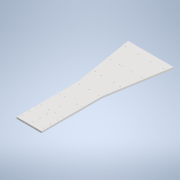
# Autodesk Inventor part: шея2,0
Saved by Autodesk Inventor 2020 (Build 240168000, 168)
## iProperties
Created: 2022-03-06
Part Number: шея2,0
Material: Типовые
Document SubType Name: Modeling
Designer: Администратор
Density: 1 g/cm^3
Appearance: По умолчанию
Author: Администратор
Autodesk Inventor part; units mm, degrees
ref_plane "YZ Plane" through (0, 0, 0) normal (1, 0, 0) x (0, 1, 0)
ref_plane "XZ Plane" through (0, 0, 0) normal (0, 1, 0) x (-1, 0, 0)
ref_plane "XY Plane" through (0, 0, 0) normal (0, 0, 1) x (1, 0, 0)
sketch "Эскиз1" plane through (0, 0, 0) normal (0, 1, 0) x (-1, 0, 0)
  line L0 (0, 0) -> (0, 458.3537) construction
  line L1 (0, 0) -> (0, -395.9132) construction
  line L2 (0, 0) -> (0, -1420) construction
  line L3 (0, -1420) -> (-240, -1420) construction
  line L4 (0, -1420) -> (240, -1420) construction
  line L5 (-240, -1420) -> (-11.5109, -68.1064) construction
  line L6 (-45, 13.7558) -> (45, 13.7558)
  line L7 (45, 13.7558) -> (45, -206.2442)
  line L8 (45, -206.2442) -> (-45, -206.2442) construction
  line L9 (-45, -206.2442) -> (-45, 13.7558)
  line L10 (-45, 13.7558) -> (45, -206.2442) construction
  line L11 (45, 13.7558) -> (-45, -206.2442) construction
  line L12 (-251.832, -1430) -> (-82.1831, -426.2442) construction
  line L13 (-45, -206.2442) -> (45, -206.2442) construction
  line L14 (45, -206.2442) -> (45, -426.2442) construction
  line L15 (45, -426.2442) -> (-45, -426.2442) construction
  line L16 (-45, -426.2442) -> (-45, -206.2442) construction
  line L17 (0, -426.2442) -> (-82.1831, -426.2442)
  line L18 (-82.1831, -426.2442) -> (-45, -206.2442)
  line L19 (0, -426.2442) -> (82.1831, -426.2442)
  line L20 (82.1831, -426.2442) -> (45, -206.2442)
  circle A0 centre (-11.5109, -68.1064) radius 1.5
  line L21 (-11.5109, -68.1064) -> (0, 0) construction
  circle A1 centre (-22.8432, -135.1555) radius 1.5
  circle A2 centre (-34.1754, -202.2045) radius 1.5
  circle A3 centre (-45.5077, -269.2536) radius 1.5
  circle A4 centre (-56.8399, -336.3027) radius 1.5
  circle A5 centre (-68.1721, -403.3518) radius 1.5
  circle A6 centre (11.5109, -68.1064) radius 1.5
  circle A7 centre (22.8432, -135.1555) radius 1.5
  circle A8 centre (34.1754, -202.2045) radius 1.5
  circle A9 centre (45.5077, -269.2536) radius 1.5
  circle A10 centre (56.8399, -336.3027) radius 1.5
  circle A11 centre (68.1721, -403.3518) radius 1.5
  line L22 (0, -96.2442) -> (0, -202.2045)
  circle A12 centre (0, -202.2045) radius 1.5
  circle A13 centre (0, -149.2045) radius 1.5
  circle A14 centre (0, -96.2045) radius 1.5
  point P0 (0, -96.2442)
  dimension "d16" = 240
  dimension "d17" = 180
  dimension "d18" = 1420
  dimension "d21" = 90
  dimension "d22" = 220
  dimension "d24" = 10
  dimension "d25" = 90
  dimension "d26" = 220
  dimension "d27" = 3
  dimension "d30" = 68
  dimension "d39" = 53
  constraints: 46 end point, 15 centre point, 7 symmetric about line, 5 horizontal, 4 midpoint, 4 parallel, 4 point on line, 4 vertical, 2 perpendicular, 1 coincident, 1 collinear, 21 other
  measures "d16" distance of L2.end L3.end
  measures "d17" angle of L3 L4
  measures "d18" distance of L0.start L2.end
  measures "d21" distance of L8.end L7.end
  measures "d22" distance of L6.end L7.end
  measures "d24" distance between parallel lines of L5 L12
  measures "d25" distance of L14.end L15.end
  measures "d26" distance of L13.end L14.end
  measures "d27" diameter of A0
  measures "d30" distance of L5.end A1.centre
  measures "d39" distance of A12.centre A13.centre
extrude "Выдавливание1" add sketch "Эскиз1" along normal blind 6 contours L6 L7 L20 L19 L17 L18 L9 | A12 | A13 L22 | L22 A13 | A14
extrude "Выдавливание2" cut sketch "Эскиз1" along normal blind 10 contours A12 | A13 L22 | L22 A13 | A14
sketch "Эскиз2" plane through (0, 6, 0) normal (0, 1, 0) x (1, 0, 0)
  circle A0 centre (-45.5077, 269.2536) radius 1.5 projected
  circle A1 centre (-56.8399, 336.3027) radius 1.5 projected
  circle A2 centre (0, 202.2045) radius 1.5 projected
  circle A3 centre (0, 149.2045) radius 1.5 projected
  circle A4 centre (0, 96.2045) radius 1.5 projected
  line L0 (45, 206.2442) -> (82.1831, 426.2442) projected
  line L1 (82.1831, 426.2442) -> (-82.1831, 426.2442) projected
  line L2 (-82.1831, 426.2442) -> (-45, 206.2442) projected
  line L3 (-45, 206.2442) -> (-45, -13.7558) projected
  line L4 (-45, -13.7558) -> (45, -13.7558) projected
  line L5 (45, -13.7558) -> (45, 206.2442) projected
  circle A5 centre (11.5109, 68.1064) radius 1.5 projected
  circle A6 centre (22.8432, 135.1555) radius 1.5 projected
  circle A7 centre (34.1754, 202.2045) radius 1.5 projected
  circle A8 centre (-11.5109, 68.1064) radius 1.5 projected
  circle A9 centre (-22.8432, 135.1555) radius 1.5 projected
  circle A10 centre (-34.1754, 202.2045) radius 1.5 projected
  circle A11 centre (45.5077, 269.2536) radius 1.5 projected
  circle A12 centre (56.8399, 336.3027) radius 1.5 projected
  circle A13 centre (68.1721, 403.3518) radius 1.5 projected
  circle A14 centre (-45.5077, 269.2536) radius 1.5 projected
  circle A15 centre (-56.8399, 336.3027) radius 1.5 projected
  circle A16 centre (-68.1721, 403.3518) radius 1.5 projected
  line L6 (-82.1831, 426.2442) -> (-45, 206.2442) projected
  line L7 (-55.6495, 269.2536) -> (55.6495, 269.2536)
  line L8 (45, 206.2442) -> (82.1831, 426.2442) projected
  line L9 (-66.9817, 336.3027) -> (66.9817, 336.3027)
  line L10 (-78.314, 403.3518) -> (78.314, 403.3518)
  circle A17 centre (-22.8432, 269.2536) radius 1.5
  circle A18 centre (22.8432, 269.2536) radius 1.5
  circle A19 centre (-22.8432, 336.3027) radius 1.5
  circle A20 centre (22.8432, 336.3027) radius 1.5
  circle A21 centre (-22.8432, 403.3518) radius 1.5
  circle A22 centre (22.8432, 403.3518) radius 1.5
  point P0 (0, 0)
  constraints: 12 point on line, 6 centre point, 6 end point, 2 parallel, 1 horizontal
extrude "Выдавливание3" cut sketch "Эскиз2" against normal blind 10 contours A17 L7 | L7 A17 | A18 L7 | L7 A18 | A19 L9 | L9 A19 | A21 L10 | L10 A21 | A20 L9 | L9 A20 | A22 L10 | L10 A22
sketch "Эскиз3" plane through (0, 6, 0) normal (0, 1, 0) x (1, 0, 0)
  circle A0 centre (-22.8432, 336.3027) radius 1.5 projected
  circle A1 centre (22.8432, 403.3518) radius 1.5 projected
  circle A2 centre (22.8432, 269.2536) radius 1.5 projected
  circle A3 centre (22.8432, 336.3027) radius 1.5 projected
  circle A4 centre (-22.8432, 403.3518) radius 1.5 projected
  circle A5 centre (-22.8432, 269.2536) radius 1.5 projected
  circle A6 centre (0, 202.2045) radius 1.5 projected
  circle A7 centre (0, 149.2045) radius 1.5 projected
  circle A8 centre (0, 96.2045) radius 1.5 projected
  line L0 (45, 206.2442) -> (82.1831, 426.2442) projected
  line L1 (82.1831, 426.2442) -> (-82.1831, 426.2442) projected
  line L2 (-82.1831, 426.2442) -> (-45, 206.2442) projected
  line L3 (-45, 206.2442) -> (-45, -13.7558) projected
  line L4 (-45, -13.7558) -> (45, -13.7558) projected
  line L5 (45, -13.7558) -> (45, 206.2442) projected
  circle A9 centre (11.5109, 68.1064) radius 1.5 projected
  circle A10 centre (22.8432, 135.1555) radius 1.5 projected
  circle A11 centre (34.1754, 202.2045) radius 1.5 projected
  circle A12 centre (-11.5109, 68.1064) radius 1.5 projected
  circle A13 centre (-22.8432, 135.1555) radius 1.5 projected
  circle A14 centre (-34.1754, 202.2045) radius 1.5 projected
  circle A15 centre (45.5077, 269.2536) radius 1.5 projected
  circle A16 centre (56.8399, 336.3027) radius 1.5 projected
  circle A17 centre (68.1721, 403.3518) radius 1.5 projected
  circle A18 centre (-45.5077, 269.2536) radius 1.5 projected
  circle A19 centre (-56.8399, 336.3027) radius 1.5 projected
  circle A20 centre (-68.1721, 403.3518) radius 1.5 projected
  line L6 (-45, 206.2442) -> (-45, -13.7558) projected
  line L7 (-45, 68.1064) -> (45, 68.1064)
  line L8 (45, -13.7558) -> (45, 206.2442) projected
  line L9 (-45, 135.1555) -> (45, 135.1555)
  circle A21 centre (-38.4, 135.1555) radius 1.5
  circle A22 centre (-38.4, 68.1064) radius 1.5
  circle A23 centre (38.4, 68.1064) radius 1.5
  circle A24 centre (38.4, 135.1555) radius 1.5
  line L10 (-39.9, 0) -> (38.4, 0)
  line L11 (0, 0) -> (0, 68.1064)
  circle A25 centre (38.4, 0) radius 1.5
  circle A26 centre (0, 0) radius 1.5
  circle A27 centre (-38.4, 0) radius 1.5
  line L12 (-39.9, 25) -> (38.4, 25)
  circle A28 centre (-38.4, 25) radius 1.5
  circle A29 centre (0, 25) radius 1.5
  circle A30 centre (38.4, 25) radius 1.5
  line L13 (-39.9, 50) -> (38.4, 50)
  circle A31 centre (-38.4, 50) radius 1.5
  circle A32 centre (0, 50) radius 1.5
  circle A33 centre (38.4, 50) radius 1.5
  dimension "d48" = 3
  dimension "d49" = 6.6
  dimension "d50" = 6.6
  dimension "d51" = 6.6
  dimension "d52" = 6.6
  dimension "d62" = 25
  constraints: 12 end point, 11 point on line, 10 centre point, 4 coincident, 3 horizontal alignment, 3 vertical, 2 horizontal, 1 midpoint, 1 perpendicular, 22 other
  measures "d48" diameter of A21
  measures "d49" distance of A22.centre L7.start
  measures "d50" distance of A21.centre L9.start
  measures "d51" distance of L7.end A23.centre
  measures "d52" distance of L9.end A24.centre
  measures "d62" distance of L10.start L12.start
extrude "Выдавливание4" cut sketch "Эскиз3" against normal blind 10 contours A33 | A30 | A25 | A27 L10 | L10 A27 | A26 L10 L11 | L11 L10 A26 | A28 L12 | L12 A28 | A29 L12 L11 | L11 L12 A29 | A31 L13 | L13 A31 | A32 L13 L11 | L11 L13 A32 | A24 L9 | L9 A24 | A23 L7 | L7 A23 | A21 L9 | L9 A21 | A22 L7 | L7 A22 | L13 A32 L11 | L11 A32 L13 | L12 A29 L11 | L11 A29 L12 | L10 A26
sketch "Эскиз4" plane through (0, 0, 0) normal (0, -1, 0) x (1, 0, 0)
  circle A0 centre (-22.8432, -336.3027) radius 1.5 projected
  circle A1 centre (22.8432, -336.3027) radius 1.5 projected
  circle A2 centre (-22.8432, -336.3027) radius 1.5 projected
  line L0 (-22.8432, -336.3027) -> (22.8432, -336.3027)
  line L1 (0, -336.3027) -> (14.75, -336.3027)
  line L2 (0, -336.3027) -> (-14.75, -336.3027)
  circle A3 centre (-14.75, -336.3027) radius 1.45
  circle A4 centre (14.75, -336.3027) radius 1.45
  point P0 (0, 0)
  dimension "d69" = 14.75
  dimension "d70" = 14.75
  dimension "d71" = 2.9
  dimension "d72" = 2.9
  constraints: 6 end point, 2 centre point, 2 coincident, 2 point on line, 1 horizontal, 1 midpoint
  measures "d69" distance of L1.start L1.end
  measures "d70" distance of L1.start L2.end
  measures "d71" diameter of A3
  measures "d72" diameter of A4
extrude "Выдавливание5" cut sketch "Эскиз4" against normal through all contours A4 L0 | L0 A4 | A3 L0 | L0 A3
